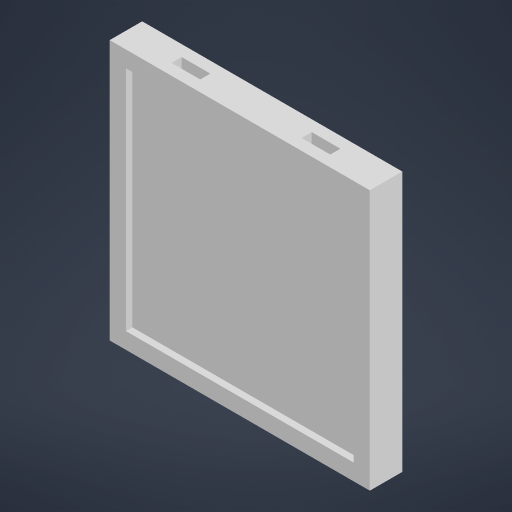
# Autodesk Inventor part: Marker_TestFit
Saved by Autodesk Inventor 2024 (Build 280153000, 153)
## iProperties
Created: 2023-07-12
Part Number: Marker_TestFit
Material: Generic
Document SubType Name: Modeling
Designer: User
Density: 1 g/cm^3
Appearance: Default
Author: User
Autodesk Inventor part; units mm, degrees
ref_plane "YZ Plane" through (0, 0, 0) normal (1, 0, 0) x (0, 1, 0)
ref_plane "XZ Plane" through (0, 0, 0) normal (0, 1, 0) x (-1, 0, 0)
ref_plane "XY Plane" through (0, 0, 0) normal (0, 0, 1) x (1, 0, 0)
sketch "Sketch1" plane through (0, 0, 0) normal (0, 0, 1) x (1, 0, 0)
  line L0 (0, 0) -> (-80, 0)
  line L1 (-80, 0) -> (-80, 80)
  line L2 (-80, 80) -> (0, 80)
  line L3 (0, 80) -> (0, 0)
  line L4 (-75, 75) -> (-5, 75)
  line L5 (-5, 75) -> (-5, 5)
  line L6 (-5, 5) -> (-75, 5)
  line L7 (-75, 5) -> (-75, 75)
  dimension "d0" = 80
  dimension "d1" = 80
  dimension "d2" = 70
  dimension "d3" = 70
  constraints: 16 end point, 4 parallel, 2 horizontal, 2 perpendicular
  measures "d0" distance of L1.end L2.end
  measures "d1" distance of L0.end L1.end
  measures "d2" distance of L5.end L6.end
  measures "d3" distance of L4.end L5.end
extrude "Extrusion1" add sketch "Sketch1" along normal blind 10 contours L0 L1 L2 L3 | L4 L5 L6 L7
sketch "Sketch2" plane through (-80, 80, 0) normal (0, 1, 0) x (1, 0, 0)
  line L0 (24.4, -3.45) -> (15.6, -3.45)
  line L1 (15.6, -3.45) -> (15.6, -6.55)
  line L2 (15.6, -6.55) -> (24.4, -6.55)
  line L3 (24.4, -6.55) -> (24.4, -3.45)
  line L4 (64.4, -3.45) -> (55.6, -3.45)
  line L5 (55.6, -3.45) -> (55.6, -6.55)
  line L6 (55.6, -6.55) -> (64.4, -6.55)
  line L7 (64.4, -6.55) -> (64.4, -3.45)
  point P0 (80, 0)
  point P1 (20, -5)
  point P2 (60, -5)
  dimension "d8" = 8.8
  dimension "d9" = 3.1
  dimension "d12" = 8.8
  dimension "d13" = 3.1
  constraints: 16 end point, 4 parallel, 2 horizontal, 2 perpendicular
  measures "d8" distance of L2.end L1.end
  measures "d9" distance of L1.end L0.end
  measures "d12" distance of L6.end L5.end
  measures "d13" distance of L5.end L4.end
extrude "Extrusion2" cut sketch "Sketch2" against normal blind 10
sketch "Sketch4" plane through (0, 0, 10) normal (0, 0, 1) x (1, 0, 0)
  line L0 (-5, 5) -> (-75, 5)
  line L1 (-75, 5) -> (-75, 75)
  line L2 (-75, 75) -> (-5, 75)
  line L3 (-5, 75) -> (-5, 5)
  point P0 (0, 0)
  dimension "d21" = 70
  dimension "d22" = 70
  constraints: 8 end point, 2 parallel, 1 horizontal, 1 perpendicular
  measures "d21" distance of L1.end L2.end
  measures "d22" distance of L0.end L1.end
extrude "Extrusion3" cut sketch "Sketch4" against normal blind 2
sketch "Sketch5" plane through (-80, 0, 0) normal (0, -1, 0) x (1, 0, 0)
  line L0 (2, 2) -> (12, 2)
  line L1 (12, 2) -> (12, 5)
  line L2 (12, 5) -> (2, 5)
  line L3 (2, 5) -> (2, 2)
  line L4 (78, 2) -> (68, 2)
  line L5 (68, 2) -> (68, 5)
  line L6 (68, 5) -> (78, 5)
  line L7 (78, 5) -> (78, 2)
  point P0 (80, 0)
  dimension "d25" = 10
  dimension "d26" = 3
  dimension "d27" = 10
  dimension "d28" = 3
  constraints: 16 end point, 4 parallel, 2 horizontal, 1 perpendicular, 2 other
  measures "d25" distance of L2.end L1.end
  measures "d26" distance of L1.end L0.end
  measures "d27" distance of L5.end L6.end
  measures "d28" distance of L4.end L5.end
extrude "Extrusion4" cut sketch "Sketch5" against normal blind 10
body "Solid1"
